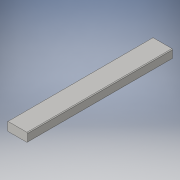
# Autodesk Inventor part: Center Support
Saved by Autodesk Inventor 2016 (Build 200138000, 138)
## iProperties
Created: 2016-07-05
Part Number: Center Support
Material: Generic
Document SubType Name: Modeling
Designer: kurti
Density: 1 g/cm^3
Appearance: Default
Author: kurti
Autodesk Inventor part; units mm, degrees
ref_plane "YZ Plane" through (0, 0, 0) normal (1, 0, 0) x (0, 1, 0)
ref_plane "XZ Plane" through (0, 0, 0) normal (0, 1, 0) x (-1, 0, 0)
ref_plane "XY Plane" through (0, 0, 0) normal (0, 0, 1) x (1, 0, 0)
sketch "Sketch1" plane through (0, 0, 0) normal (0, 0, 1) x (1, 0, 0)
  line L0 (-44.45, 19.05) -> (44.45, 19.05)
  line L1 (44.45, 19.05) -> (44.45, -19.05)
  line L2 (44.45, -19.05) -> (-44.45, -19.05)
  line L3 (-44.45, -19.05) -> (-44.45, 19.05)
  line L4 (-44.45, 19.05) -> (44.45, -19.05) construction
  line L5 (44.45, 19.05) -> (-44.45, -19.05) construction
  point P0 (0, 0)
  dimension "d0" = 88.9
  dimension "d1" = 38.1
  constraints: 12 end point, 2 midpoint, 2 parallel, 1 horizontal, 1 perpendicular
  measures "d0" distance of L1.end L2.end
  measures "d1" distance of L0.end L1.end
extrude "Extrusion1" add sketch "Sketch1" along normal blind 635
fillet "Fillet1" radius 3.175 4 edges at (-44.45, -19.05, 317.5) (-44.45, 19.05, 317.5) (44.45, 19.05, 317.5) (44.45, -19.05, 317.5)
body "Solid1"
